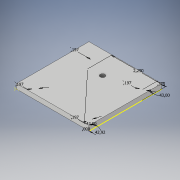
# Autodesk Inventor part: plateform
Saved by Autodesk Inventor 2017 (Build 210142000, 142)
## iProperties
Created: 2018-11-16
Part Number: plateform
Material: Generic
Document SubType Name: Modeling
Designer: Antoine Blaud
Density: 1 g/cm^3
Appearance: Default
Author: Antoine Blaud
Autodesk Inventor part; units mm, degrees
ref_plane "YZ Plane" through (0, 0, 0) normal (1, 0, 0) x (0, 1, 0)
ref_plane "XZ Plane" through (0, 0, 0) normal (0, 1, 0) x (-1, 0, 0)
ref_plane "XY Plane" through (0, 0, 0) normal (0, 0, 1) x (1, 0, 0)
sketch "Sketch1" plane through (0, 0, 0) normal (1, 0, 0) x (0, 1, 0)
  line L0 (0, 0) -> (10, 0)
  line L1 (10, 0) -> (10, -20)
  line L2 (10, -20) -> (0, -20)
  line L3 (0, -20) -> (0, 0)
  circle A0 centre (5, 0) radius 3.81
  circle A1 centre (5, -20) radius 3.81
  line L4 (10, 0) -> (0, 0)
  line L5 (0, 0) -> (0, 7.62)
  line L6 (0, 7.62) -> (10, 7.62)
  line L7 (10, 7.62) -> (10, 0)
  line L8 (0, -20) -> (10, -20)
  line L9 (10, -20) -> (10, -27.62)
  line L10 (10, -27.62) -> (0, -27.62)
  line L11 (0, -27.62) -> (0, -20)
  dimension "d0" = 10
  dimension "d1" = 20
  dimension "d2" = 7.62
  dimension "d3" = 7.62
  dimension "d4" = 10
  dimension "d5" = 7.62
  dimension "d7" = 7.62
  constraints: 24 end point, 6 parallel, 3 horizontal, 3 perpendicular, 2 centre point, 2 midpoint, 1 point on line
  measures "d0" distance between parallel lines of L1 L3
  measures "d1" distance between parallel lines of L0 L2
  measures "d2" diameter of A0
  measures "d3" diameter of A1
  measures "d4" distance between parallel lines of L5 L1
  measures "d5" distance between parallel lines of L6 L4
  measures "d7" distance of L10.end L2.end
extrude "Extrusion1" add sketch "Sketch1" along normal blind 38.1
extrude "Extrusion2" cut sketch "Sketch1" along normal blind 38.1 contours A0 L0 | L0 A0 | A1 L2 | L2 A1
sketch "Sketch2" plane through (0, 10, 7.62) normal (0, 1, 0) x (1, 0, 0)
  line L0 (57.15, -20.4851) -> (-19.05, -20.4851)
  line L1 (-19.05, -20.4851) -> (-19.05, 55.7149)
  line L2 (-19.05, 55.7149) -> (57.15, 55.7149)
  line L3 (57.15, 55.7149) -> (57.15, -20.4851)
  line L4 (57.15, -20.4851) -> (-19.05, 55.7149) construction
  line L5 (-19.05, -20.4851) -> (57.15, 55.7149) construction
  line L6 (0, 0) -> (38.1, 0) projected
  line L7 (0, 35.24) -> (38.1, 35.24) projected
  line L8 (-19.05, 17.6149) -> (4.7227, 17.6149)
  line L9 (57.15, 17.6149) -> (33.3773, 17.6149)
  circle A0 centre (4.7227, 17.6149) radius 2.5
  circle A1 centre (33.3773, 17.6149) radius 2.5
  line L10 (19.05, 55.7149) -> (19.05, 31.9422)
  circle A2 centre (19.05, 31.9422) radius 2.5
  point P0 (0, 7.62)
  point P1 (19.05, 17.6149)
  dimension "d12" = 17.6149
  dimension "d13" = 17.6251
  dimension "d14" = 35.24
  dimension "d15" = 76.2
  dimension "d16" = 76.2
  dimension "d17" = 19.05
  dimension "d32" = 23.7727
  dimension "d33" = 23.7727
  dimension "d34" = 5
  dimension "d35" = 5
  dimension "d38" = 23.7727
  dimension "d39" = 5
  constraints: 18 end point, 5 midpoint, 3 centre point, 3 coincident, 3 horizontal, 2 parallel, 1 perpendicular, 1 vertical
  measures "d12" distance from line of L6 point (19.05, 17.615)
  measures "d13" distance from line of L7 point (19.05, 17.615)
  measures "d14" distance between parallel lines of L7 L6
  measures "d15" distance of L2.end L0.start
  measures "d16" distance of L1.end L2.end
  measures "d17" distance from line of L7.end L3
  measures "d32" distance of L8.start L8.end
  measures "d33" distance of L9.start L9.end
  measures "d34" diameter of A1
  measures "d35" diameter of A0
  measures "d38" distance of L10.start L10.end
  measures "d39" diameter of A2
extrude "Extrusion3" add sketch "Sketch2" along normal blind 5 contours L0 L1 L2 L3 | A0 | A1 | A2
sketch "Sketch3" plane through (0, 10, 7.62) normal (0, -1, 0) x (1, 0, 0)
  line L0 (0, 0) -> (38.1, 0) projected
  line L1 (0, 0) -> (-19.05, 20.4851)
  line L2 (-19.05, 20.4851) -> (-19.05, -55.7149) projected
  line L3 (-19.05, -55.7149) -> (0, -35.2882)
  line L4 (57.15, -55.7149) -> (57.15, 20.4851) projected
  line L5 (57.15, -55.7149) -> (38.1, -35.2882)
  line L6 (38.1, 0) -> (57.15, 20.4851)
  circle A0 centre (47.625, -45.5015) radius 2.5
  circle A1 centre (47.625, 10.2425) radius 2.5
  circle A2 centre (-9.525, -45.5015) radius 2.5
  circle A3 centre (-9.525, 10.2425) radius 2.5
  point P0 (0, -7.62)
  dimension "d20" = 5
  dimension "d21" = 5
  dimension "d22" = 5
  dimension "d23" = 5
  dimension "d24" = 42.921
  dimension "d25" = 43.003
  dimension "d26" = 43.003
  dimension "d27" = 0
  dimension "d28" = 9.525
  dimension "d29" = 57.15
  constraints: 8 end point, 4 centre point, 4 midpoint
  measures "d20" diameter of A0
  measures "d21" diameter of A1
  measures "d22" diameter of A2
  measures "d23" diameter of A3
  measures "d24" angle of L4 L6
  measures "d25" angle of L4 L5
  measures "d26" angle of L4 L3
  measures "d27" distance from line of L6.end L4
  measures "d28" distance from line of A0.centre L4
  measures "d29" distance from line of L3.end L4
extrude "Extrusion4" cut sketch "Sketch3" against normal blind 2
extrude "Extrusion6" cut sketch "Sketch2" along normal mid plane 25.4 contours A2
thread "Thread1" size "M1x0.25" class "6H" standard "ISO Metric profile" full length
body "Solid1"
